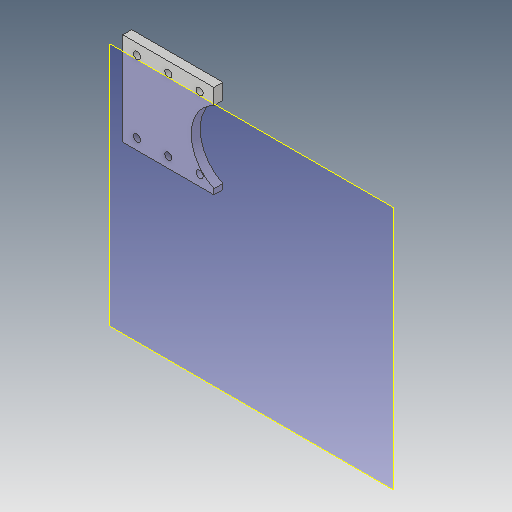
# Autodesk Inventor part: 02_Zeiss_Axiotech_adapterplate_rightleft_connector
Saved by Autodesk Inventor 2019 (Build 230136000, 136)
## iProperties
Created: 2019-05-07
Part Number: 02_Zeiss_Axiotech_adapterplate_rightleft_connector
Material: Generic
Document SubType Name: Modeling
Designer: diederichbenedict
Density: 1 g/cm^3
Appearance: Default
Author: diederichbenedict
Autodesk Inventor part; units mm, degrees
ref_plane "YZ Plane" through (0, 0, 0) normal (1, 0, 0) x (0, 1, 0)
ref_plane "XZ Plane" through (0, 0, 0) normal (0, 1, 0) x (-1, 0, 0)
ref_plane "XY Plane" through (0, 0, 0) normal (0, 0, 1) x (1, 0, 0)
ref_plane "Work Plane2" through (153.4386, -53.4776, -92.0146) normal (0, 0, -1) x (0, -1, 0)
sketch "Sketch2" plane through (153.4386, -53.4776, -92.0146) normal (0, 0, -1) x (0, -1, 0)
  line L0 (93.2, 97.5) -> (213.5, 97.5) construction
  line L1 (40, 105.5) -> (170, 105.5) construction
  line L2 (-3.5, 97.5) -> (93.2, 97.5) construction
  line L3 (40, 105.5) -> (170, 105.5) construction
  line L4 (0.0695, 95.5) -> (93.2, 95.5) construction
  line L5 (93.2, 95.5) -> (209.9305, 95.5) construction
  arc A0 (93.2, 56.229) -> (86.5748, 48.5) centre (107.9, 36.9243) ccw construction
  line L6 (93.2, 95.5) -> (93.2, 56.229) construction
  arc A1 (120.0681, 57.9171) -> (93.2, 56.229) centre (107.9, 36.9243) ccw construction
  arc A2 (128.5511, 49.6637) -> (120.0681, 57.9171) centre (125, 54.5) ccw construction
  arc A3 (129.2252, 48.5) -> (128.5511, 49.6637) centre (107.9, 36.9243) ccw construction
  line L7 (134.8038, 48.5) -> (129.2252, 48.5) construction
  arc A4 (145.1962, 48.5) -> (134.8038, 48.5) centre (140, 51.5) ccw construction
  line L8 (159.8038, 48.5) -> (145.1962, 48.5) construction
  arc A5 (170.1962, 48.5) -> (159.8038, 48.5) centre (165, 51.5) ccw construction
  line L9 (184.8038, 48.5) -> (170.1962, 48.5) construction
  arc A6 (195.1962, 48.5) -> (184.8038, 48.5) centre (190, 51.5) ccw construction
  line L10 (198.5, 48.5) -> (195.1962, 48.5) construction
  arc A7 (204.5, 42.5) -> (198.5, 48.5) centre (198.5, 42.5) ccw construction
  line L11 (204.5, -42.5) -> (204.5, 42.5) projected
  arc A8 (204.5, -42.5) -> (206.5, -44.5) centre (206.5, -42.5) ccw projected
  line L12 (207.3038, -44.5) -> (206.5, -44.5) projected
  arc A9 (215.5, -36.3038) -> (207.3038, -44.5) centre (212.5, -41.5) ccw projected
  line L13 (215.5, 87.3038) -> (215.5, -36.3038) construction
  arc A10 (207.3038, 95.5) -> (215.5, 87.3038) centre (212.5, 92.5) ccw construction
  line L14 (125, 95.5) -> (207.3038, 95.5) construction
  circle A11 centre (125, 89.5) radius 6 construction
  line L15 (93.2, 95.5) -> (125, 95.5) construction
  circle A12 centre (125, 72) radius 6 construction
  circle A13 centre (190, 76.5) radius 6 construction
  circle A14 centre (140, 76.5) radius 6 construction
  arc A15 (93.2, 53.646) -> (87.8, 46.5) centre (107.9, 36.9243) ccw construction
  arc A16 (128, 46.5) -> (93.2, 53.646) centre (107.9, 36.9243) ccw construction
  circle A17 centre (85, 89.5) radius 6 construction
  circle A18 centre (125, 89.5) radius 6 construction
  line L16 (79, 97.5) -> (79, 46.5)
  line L17 (79, 46.5) -> (87.8, 46.5)
  line L18 (79, 97.5) -> (131, 97.5)
  line L19 (131, 97.5) -> (131, 48.5)
  line L20 (131, 48.5) -> (131, 46.5)
  line L21 (131, 46.5) -> (128, 46.5)
  arc A19 (128, 46.5) -> (87.8, 46.5) centre (107.9, 36.9243) ccw
  circle A20 centre (85, 54.5) radius 1.95 projected
  circle A21 centre (85, 72) radius 1.95 projected
  circle A22 centre (85, 89.5) radius 1.95 projected
  circle A23 centre (125, 89.5) radius 1.95 projected
  circle A24 centre (125, 72) radius 1.95 projected
  circle A25 centre (125, 54.5) radius 1.95 projected
  point P0 (-53.4776, 153.4386)
  constraints: 12 end point, 4 point on line, 3 perpendicular, 2 point on circle, 2 vertical alignment, 1 centre point, 1 concentric, 1 vertical
extrude "Extrusion2" add sketch "Sketch2" along normal blind 5
shell "Shell2" thickness 2 removed faces 1 at (70.074, -152.3865, -97.0146)
body "Solid2"
